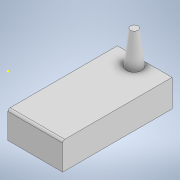
# Autodesk Inventor part: kappale
Saved by Autodesk Inventor 2020.1 (Build 241239000, 239)
## iProperties
Created: 2021-11-08
Part Number: kappale
Material: Generic
Document SubType Name: Modeling
Designer: s1mate03
Density: 1 g/cm^3
Appearance: Default
Author: s1mate03
Autodesk Inventor part; units mm, degrees
ref_plane "YZ Plane" through (0, 0, 0) normal (1, 0, 0) x (0, 1, 0)
ref_plane "XZ Plane" through (0, 0, 0) normal (0, 1, 0) x (-1, 0, 0)
sketch "Sketch1" plane through (0, 0, 0) normal (0, 1, 0) x (-1, 0, 0)
  line L0 (0, 0) -> (-50, 0)
  line L1 (-50, 0) -> (-50, -100)
  line L2 (-50, -100) -> (0, -100)
  line L3 (0, -100) -> (0, 0)
  dimension "d3" = 100
  dimension "d4" = 50
  constraints: 8 end point, 2 parallel, 1 horizontal, 1 perpendicular
  measures "d3" distance of L0.end L1.end
  measures "d4" distance of L1.end L2.end
extrude "Extrusion1" add sketch "Sketch1" along normal blind 25
fillet "Fillet1" radius 2 1 edges at (25, 25, 0)
ref_plane "Work Plane1" through (0, 55, 0) normal (0, 1, 0) x (1, 0, 0)
sketch "Sketch2" plane through (0, 55, 0) normal (0, 1, 0) x (1, 0, 0)
  point P0 (0, 0)
sketch "Sketch3" plane through (0, 25, 0) normal (0, 1, 0) x (1, 0, 0)
  circle A0 centre (23.7799, 91.5707) radius 6.9252
  point P0 (0, 0)
  constraints: 1 centre point
sketch "Sketch4" plane through (0, 55, 0) normal (0, 1, 0) x (1, 0, 0)
  circle A0 centre (23.7424, 91.7378) radius 3.5123
  point P0 (0, 0)
  constraints: 1 centre point
loft "Loft1" add profiles "Sketch3", "Sketch4"
sketch "Sketch5" plane through (0, 0, 0) normal (0, -1, 0) x (1, 0, 0)
  line L0 (50, -100) -> (0, -100) projected
  line L1 (50, -100) -> (50, -90)
  line L2 (50, -2) -> (50, -100) projected
  line L3 (50, -90) -> (40, -90)
  circle A0 centre (40, -90) radius 2.5
  line L4 (40, -90) -> (40, -73.1599)
  line L5 (40, -90) -> (17.7006, -90)
  circle A1 centre (40, -70) radius 2.5
  circle A2 centre (40, -50) radius 2.5
  circle A3 centre (20, -90) radius 2.5
  circle A4 centre (20, -70) radius 2.5
  circle A5 centre (20, -50) radius 2.5
  point P0 (0, 0)
  dimension "d10" = 10
  dimension "d11" = 10
  dimension "d12" = 5
  dimension "d15" = 20
  dimension "d18" = 20
  constraints: 8 end point, 6 centre point, 2 horizontal, 2 vertical, 1 coincident, 1 perpendicular, 1 point on line, 10 other
  measures "d10" distance of L0.start L1.end
  measures "d11" distance of L1.end L3.end
  measures "d12" diameter of A0
  measures "d15" distance of L4.start A1.centre
  measures "d18" distance of L4.start A3.centre
extrude "Extrusion2" cut sketch "Sketch5" against normal blind 5
body "Solid1"
